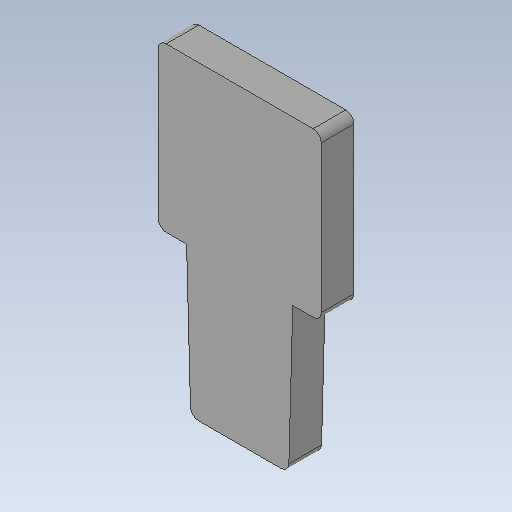
# Autodesk Inventor part: hage
Saved by Autodesk Inventor 2020.1 (Build 241239000, 239)
## iProperties
Created: 2019-10-04
Part Number: hage
Material: S235JR
Document SubType Name: Sheet Metal
Designer: gust3763
Density: 7.85 g/cm^3
Flat Pattern Width: 7.6 cm
Flat Pattern Length: 4 cm
Flat Pattern Area: 30.4 cm^2
Sheet Metal Rule: Default_mm
Sheet Metal Width: 76,000 mm
Sheet Metal Length: 40,000 mm
Sheet Metal Area: 3040,000 mm^2
Appearance: Light Gray
Author: gust3763
Autodesk Inventor part; units mm, degrees
ref_plane "YZ Plane" through (0, 0, 0) normal (1, 0, 0) x (0, 1, 0)
ref_plane "XZ Plane" through (0, 0, 0) normal (0, 1, 0) x (-1, 0, 0)
ref_plane "XY Plane" through (0, 0, 0) normal (0, 0, 1) x (1, 0, 0)
sketch "Sketch1" plane through (0, 0, 0) normal (0, 0, 1) x (1, 0, 0)
  line L0 (0, 0) -> (0, 17.1478) construction
  line L1 (-10.0548, 0.1113) -> (10.0548, 0.1113)
  line L2 (12.054, 2.0558) -> (13, 36.1113)
  line L3 (13, 36.1113) -> (18, 36.1113)
  line L4 (20, 38.1113) -> (20, 74.1113)
  line L5 (18, 76.1113) -> (-18, 76.1113)
  line L6 (-20, 74.1113) -> (-20, 38.1113)
  line L7 (-18, 36.1113) -> (-13, 36.1113)
  line L8 (-13, 36.1113) -> (-12.054, 2.0558)
  arc A0 (-18, 76.1113) -> (-20, 74.1113) centre (-18, 74.1113) ccw
  arc A1 (20, 74.1113) -> (18, 76.1113) centre (18, 74.1113) ccw
  arc A2 (-20, 38.1113) -> (-18, 36.1113) centre (-18, 38.1113) ccw
  arc A3 (18, 36.1113) -> (20, 38.1113) centre (18, 38.1113) ccw
  arc A4 (-12.054, 2.0558) -> (-10.0548, 0.1113) centre (-10.0548, 2.1113) ccw
  arc A5 (10.0548, 0.1113) -> (12.054, 2.0558) centre (10.0548, 2.1113) ccw
  point P0 (-12, 0.1113)
  point P1 (12, 0.1113)
  point P2 (20, 36.1113)
  point P3 (20, 76.1113)
  point P4 (-20, 76.1113)
  dimension "d0" = 24
  dimension "d1" = 26
  dimension "d2" = 40
  dimension "d3" = 36
  dimension "d4" = 40
  dimension "d5" = 2
  measures "d0" distance of point (-12, 0.111) point (12, 0.111)
  measures "d1" distance of L2.end L7.end
  measures "d2" distance of point (20, 76.111) point (-20, 76.111)
  measures "d3" distance between parallel lines of L1 L3
  measures "d4" distance of point (20, 36.111) point (20, 76.111)
  measures "d5" radius of A0
extrude "Plate1" add sketch "Sketch1" along normal blind 8
equation "\"d6\" = Thickness"
equation "\"BendRadius\" = Thickness"
equation "\"BendReliefWidth\" = Thickness"
equation "\"BendReliefDepth\" = 0.5 * Thickness"
equation "\"CornerReliefSize\" = 4 * Thickness"
equation "\"MinimumRemnant\" = 2 * Thickness"
equation "\"TransitionRadius\" = BendRadius"
equation "\"JacobiRadiusSize\" = BendRadius"
equation "\"GapSize\" = Thickness"
equation "\"Thickness\" = 8"
body "Solid1"
